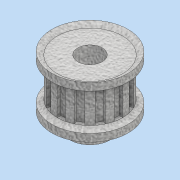
# Autodesk Inventor part: Koło zębate 21 T5 14 2F
Saved by Autodesk Inventor 2018 (Build 220112000, 112)
## iProperties
Created: 2019-01-25
Part Number: Koło zębate 21 T5 14 2F
Material: Ogólny
Document SubType Name: Modeling
Designer: Dawid
Density: 1 g/cm^3
Appearance: Aluminium odlewane
Author: Dawid
Autodesk Inventor part; units mm, degrees
ref_plane "YZ Plane" through (0, 0, 0) normal (1, 0, 0) x (0, 1, 0)
ref_plane "XZ Plane" through (0, 0, 0) normal (0, 1, 0) x (-1, 0, 0)
ref_plane "XY Plane" through (0, 0, 0) normal (0, 0, 1) x (1, 0, 0)
sketch "Szkic1" plane through (0, 0, 0) normal (0, 0, 1) x (1, 0, 0)
  arc A0 (2.3865, 10.4561) -> (0, 10.725) centre (0, 0) ccw
  arc A1 (0, 9.525) -> (2.1195, 9.2862) centre (0, 0) ccw
  line L0 (0, 9.525) -> (0, 10.725)
  line L1 (2.1195, 9.2862) -> (2.3865, 10.4561)
  constraints: 4 end point, 4 point on circle, 2 centre point, 2 coincident, 1 vertical
extrude "Wyciągnięcie proste1" add sketch "Szkic1" along normal blind 15
pattern_circular "Szyk kołowy1" count 14 over 360 about axis through (0, 0, 0) along (0, 0, 1) of "Wyciągnięcie proste1"
sketch "Szkic2" plane through (0, 0, 0) normal (0, 0, -1) x (-1, 0, 0)
  circle A0 centre (0, 0) radius 6.5
  dimension "d8" = 13
  constraints: 1 centre point, 1 coincident
  measures "d8" diameter of A0
extrude "Wyciągnięcie proste2" add sketch "Szkic2" along normal blind 6
sketch "Szkic3" plane through (0, 0, 0) normal (1, 0, 0) x (0, 1, 0)
  line L0 (0, 15) -> (-2.1195, 15) projected
  line L1 (0, 15) -> (10.725, 15)
  line L2 (12.5, 15) -> (12.5, 13.5)
  line L3 (10.725, 12.5) -> (0, 12.5)
  line L4 (0, 12.5) -> (0, 15)
  line L5 (6.5, 0) -> (-6.5, 0) projected
  line L6 (12.5, 0) -> (12.5, 1.5)
  line L7 (10.725, 2.5) -> (0, 2.5)
  line L8 (0, 0) -> (0, 15) projected
  line L9 (0, 0) -> (0, 2.5)
  line L10 (12.5, 0) -> (12.5, -1)
  line L11 (9.525, 0) -> (10.725, 0) projected
  line L12 (10.725, 0) -> (12.5, -1)
  line L13 (12.5, 1.5) -> (10.725, 2.5)
  line L14 (10.725, 0) -> (0, 0)
  line L15 (12.5, 15) -> (12.5, 16)
  line L16 (10.725, 15) -> (12.5, 16)
  line L17 (10.725, 12.5) -> (12.5, 13.5)
  point P0 (0, 0)
  constraints: 28 end point, 5 perpendicular, 2 point on line, 2 vertical, 1 collinear, 1 horizontal
revolve "Obrót1" add sketch "Szkic3" angle 360 about axis through (0, 0, 0) along (0, 0, 1)
sketch "Szkic4" plane through (0, 0, -6) normal (0, 0, -1) x (-1, 0, 0)
  circle A0 centre (0, 0) radius 4
  dimension "d22" = 8
  constraints: 1 centre point, 1 coincident
  measures "d22" diameter of A0
extrude "Wyciągnięcie proste3" cut sketch "Szkic4" against normal up to next
sketch "Szkic5" plane through (0, 0, 0) normal (0, 1, 0) x (-1, 0, 0)
  line L0 (-12.5, -1) -> (12.5, -1) projected
  line L1 (-6.5, -6) -> (6.5, -6) projected
  line L2 (6.5, 0) -> (6.5, -6) projected
  line L3 (-6.5, 0) -> (-6.5, -6) projected
  line L4 (6.5, -6) -> (-6.5, -1)
  line L5 (6.5, -1) -> (-6.5, -6)
  circle A0 centre (0, -3.5) radius 1.5
  point P0 (0, 0)
  dimension "d25" = 3
  constraints: 4 end point, 4 point on line, 1 centre point, 1 midpoint
  measures "d25" diameter of A0
extrude "Wyciągnięcie proste4" cut sketch "Szkic5" along normal up to next contours A0 L5 L4 | L4 L5 A0 | A0 L4 L5 | L5 L4 A0
thread "Gwint1" size "M3x0.5" class "6H" standard "ANSI Metric M Profile" full length
